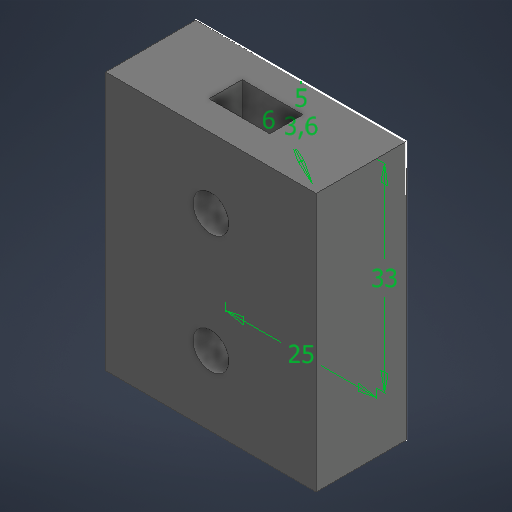
# Autodesk Inventor part: LoadCellBase
Saved by Autodesk Inventor 2027 (Build 310192000, 192)
## iProperties
Created: 2026-10-06
Part Number: LoadCellBase
Material: Genérico
Document SubType Name: Modeling
Designer: EspacoMaker
Density: 1 g/cm^3
Appearance: Padrão
Author: EspacoMaker
Autodesk Inventor part; units mm, degrees
ref_plane "YZ Plane" through (0, 0, 0) normal (1, 0, 0) x (0, 1, 0)
ref_plane "XZ Plane" through (0, 0, 0) normal (0, 1, 0) x (-1, 0, 0)
ref_plane "XY Plane" through (0, 0, 0) normal (0, 0, 1) x (1, 0, 0)
sketch "Esboço1" plane through (0, 0, 0) normal (0, 0, 1) x (1, 0, 0)
  line L0 (-12.5, 16.5) -> (12.5, 16.5) construction
  line L1 (12.5, 16.5) -> (12.5, -16.5) construction
  line L2 (12.5, -16.5) -> (-12.5, -16.5) construction
  line L3 (-12.5, -16.5) -> (-12.5, 16.5) construction
  line L4 (-12.5, 16.5) -> (12.5, -16.5) construction
  line L5 (12.5, 16.5) -> (-12.5, -16.5) construction
  line L6 (0, 16.5) -> (0, -16.5) construction
  line L7 (-12.5, 12.9) -> (12.5, 12.9) construction
  circle A0 centre (0, 9.9) radius 3
  line L8 (-12.5, 0) -> (12.5, 0) construction
  circle A1 centre (0, -9.9) radius 3
  line L9 (17.5, 21.5) -> (-17.5, 21.5)
  line L10 (-17.5, 21.5) -> (-17.5, -21.5)
  line L11 (-17.5, -21.5) -> (17.5, -21.5)
  line L12 (17.5, -21.5) -> (17.5, 21.5)
  line L13 (3, 12.9) -> (3, 0) construction
  line L14 (-3, 6.9) -> (3, 6.9) construction
  line L15 (3, 6.9) -> (3, 12.9) construction
  line L16 (3, 12.9) -> (-3, 12.9) construction
  line L17 (-3, 12.9) -> (-3, 6.9) construction
  line L18 (-3, 6.9) -> (3, 12.9) construction
  line L19 (3, 6.9) -> (-3, 12.9) construction
  point P0 (0, 0)
  dimension "d0" = 25
  dimension "d1" = 33
  dimension "d2" = 3.6
  dimension "d3" = 6
  dimension "d4" = 5
  constraints: 40 end point, 8 midpoint, 7 parallel, 4 perpendicular, 3 point on line, 2 centre point, 2 horizontal, 2 tangent, 1 symmetric about line, 4 other
  measures "d0" distance of L1.end L2.end
  measures "d1" distance of L0.end L1.end
  measures "d2" distance between parallel lines of L0 L7
  measures "d3" diameter of A0
  measures "d4" distance between parallel lines of L0 L9
extrude "Extrusão1" add sketch "Esboço1" along normal blind 15 contours A0 | A1 | L12 L11 L10 L9
sketch "Esboço3" plane through (-17.5, 21.5, 0) normal (0, 1, 0) x (1, 0, 0)
  line L0 (35, 0) -> (0, 0) projected
  line L1 (0, 0) -> (0, -15) projected
  line L2 (35, -15) -> (0, -15) projected
  line L3 (35, 0) -> (35, -15) projected
  line L4 (17.5, -15) -> (17.5, 0) construction
  line L5 (0, -7.5) -> (35, -7.5) construction
  line L6 (12.45, -4.75) -> (22.55, -4.75)
  line L7 (22.55, -4.75) -> (22.55, -10.25)
  line L8 (22.55, -10.25) -> (12.45, -10.25)
  line L9 (12.45, -10.25) -> (12.45, -4.75)
  line L10 (12.45, -4.75) -> (22.55, -10.25) construction
  line L11 (22.55, -4.75) -> (12.45, -10.25) construction
  point P0 (17.5, -7.5)
  dimension "d12" = 10.1
  dimension "d13" = 5.5
  constraints: 16 end point, 6 midpoint, 2 parallel, 2 perpendicular, 1 horizontal
  measures "d12" distance of L7.end L8.end
  measures "d13" distance of L6.end L7.end
extrude "Extrusão2" cut sketch "Esboço3" against normal blind 17 contours L6 L7 L8 L9
sketch "Esboço4" plane through (-17.5, -21.5, 0) normal (0, -1, 0) x (1, 0, 0)
  line L0 (35, 0) -> (35, 15) projected
  line L1 (35, 7.5) -> (0, 7.5) construction
  line L2 (0, 0) -> (0, 15) projected
  line L3 (17.5, 0) -> (17.5, 15) construction
  line L4 (35, 15) -> (0, 15) projected
  line L5 (22.55, 5) -> (12.45, 5)
  line L6 (12.45, 5) -> (12.45, 10)
  line L7 (12.45, 10) -> (22.55, 10)
  line L8 (22.55, 10) -> (22.55, 5)
  line L9 (22.55, 5) -> (12.45, 10) construction
  line L10 (12.45, 5) -> (22.55, 10) construction
  point P0 (17.5, 7.5)
  dimension "d16" = 10.1
  dimension "d17" = 5
  constraints: 16 end point, 6 midpoint, 2 parallel, 1 horizontal, 1 perpendicular
  measures "d16" distance of L6.end L7.end
  measures "d17" distance of L5.end L6.end
extrude "Extrusão3" cut sketch "Esboço4" against normal blind 17
extrude "Extrusão4" cut sketch "Esboço1" along normal blind 15 contours A0 | A1
